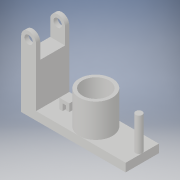
# Autodesk Inventor part: ValveBaseMk2.4
Saved by Autodesk Inventor 2019 (Build 230136000, 136)
## iProperties
Created: 2019-01-19
Part Number: ValveBaseMk2.4
Material: Generic
Document SubType Name: Modeling
Designer: Kepler
Density: 1 g/cm^3
Appearance: Default
Author: Kepler
Autodesk Inventor part; units mm, degrees
ref_plane "YZ Plane" through (0, 0, 0) normal (1, 0, 0) x (0, 1, 0)
ref_plane "XZ Plane" through (0, 0, 0) normal (0, 1, 0) x (-1, 0, 0)
ref_plane "XY Plane" through (0, 0, 0) normal (0, 0, 1) x (1, 0, 0)
sketch "Sketch1" plane through (0, 0, 0) normal (0, 0, 1) x (1, 0, 0)
  line L0 (0, 0) -> (0, 40)
  line L1 (0, 0) -> (63, 0)
  line L2 (63, 0) -> (63, 5)
  line L3 (63, 5) -> (9, 5)
  arc A0 (9, 40) -> (0, 40) centre (4.5, 40) ccw
  line L4 (9, 40) -> (9, 5)
  circle A1 centre (4.5, 40) radius 2.5
  dimension "d0" = 40
  dimension "d2" = 5
  dimension "d6" = 4.5
  dimension "d7" = 5
  dimension "d8" = 9
  dimension "d9" = 54
  dimension "d47" = 32.5
  constraints: 10 end point, 3 perpendicular, 2 centre point, 2 point on circle, 2 tangent, 1 coincident, 1 horizontal, 1 vertical
  measures "d0" distance of L0.start L0.end
  measures "d2" distance of L1.end L2.end
  measures "d6" radius of A0
  measures "d7" diameter of A1
  measures "d8" distance between parallel lines of L4 L0
  measures "d9" distance of L2.end L3.end
  measures "d47" distance edge to line of A1 L3
extrude "Extrusion1" add sketch "Sketch1" along normal blind 20
sketch "Sketch2" plane through (9, 5, 0) normal (0, 1, 0) x (1, 0, 0)
  line L0 (0, 0) -> (0, -20) projected
  circle A0 centre (26, -10) radius 10
  line L1 (0, 0) -> (54, 0) projected
  circle A1 centre (52, -10) radius 2
  line L2 (54, 0) -> (54, -20) projected
  point P0 (-9, 0)
  dimension "d14" = 20
  dimension "d16" = 26
  dimension "d20" = 4
  dimension "d21" = 10
  dimension "d22" = 14
  constraints: 2 centre point, 2 tangent
  measures "d14" diameter of A0
  measures "d16" distance from line of A0.centre L0
  measures "d20" diameter of A1
  measures "d21" distance from line of L1 A1.centre
sketch "Sketch7" plane through (9, 5, 0) normal (1, 0, 0) x (0, 0, -1)
  line L0 (-10, 41.0364) -> (-10, 39.6436)
  line L1 (0, 39.5) -> (-20, 39.5) projected
  line L2 (-2.5, 39.5) -> (-2.5, 25.5)
  line L3 (-17.5, 39.5) -> (-17.5, 25.5)
  line L4 (-17.5, 39.5) -> (-2.5, 39.5)
  line L5 (0, 32.5) -> (-20, 32.5) projected
  line L6 (-17.5, 25.5) -> (-2.5, 25.5)
  point P0 (0, -5)
  dimension "d40" = 14
  dimension "d41" = 14
  dimension "d42" = 15
  constraints: 10 end point, 2 point on line, 2 vertical, 1 collinear, 1 perpendicular, 1 other
  measures "d40" distance of L2.start L2.end
  measures "d41" distance of L3.start L3.end
  measures "d42" distance between parallel lines of L3 L2
extrude "Extrusion5" cut sketch "Sketch7" against normal blind 14
extrude "Extrusion6" add sketch "Sketch2" along normal blind 20
sketch "Sketch9" plane through (35, 25, 10) normal (0, 1, 0) x (1, 0, 0)
  circle A0 centre (0, 0) radius 8
  point P0 (-35, 10)
  dimension "d50" = 16
  constraints: 1 centre point
  measures "d50" diameter of A0
extrude "Extrusion7" cut sketch "Sketch9" against normal blind 25
sketch "Sketch10" plane through (9, 5, 20) normal (0, 1, 0) x (1, 0, 0)
  line L0 (6, 8) -> (12, 8)
  line L1 (12, 8) -> (12, 12)
  line L2 (12, 12) -> (6, 12)
  line L3 (6, 12) -> (6, 8)
  line L4 (26, 0) -> (0, 0) projected
  line L5 (0, 2.5) -> (0, 17.5) projected
  point P0 (-9, 20)
  dimension "d53" = 6
  dimension "d54" = 4
  dimension "d55" = 8
  dimension "d56" = 6
  constraints: 8 end point, 3 perpendicular, 1 horizontal
  measures "d53" distance of L0.start L0.end
  measures "d54" distance of L0.end L1.end
  measures "d55" distance between parallel lines of L4 L0
  measures "d56" distance between parallel lines of L5 L3
extrude "Extrusion8" add sketch "Sketch10" along normal blind 6
sketch "Sketch11" plane through (21, 5, 8) normal (0, 0, -1) x (-1, 0, 0)
  line L0 (2, 4) -> (4, 4)
  line L1 (6, 0) -> (6, 6) projected
  line L2 (12, 0) -> (-14, 0) projected
  line L3 (0, 0) -> (6, 0)
  line L4 (0, 1.5) -> (0, 0)
  line L5 (6, 0) -> (0, 0)
  line L6 (0, 0) -> (3, 0)
  line L7 (0, 1.5) -> (2, 1.5)
  line L8 (2, 1.5) -> (2, 4)
  line L9 (3, 0) -> (0, 0)
  line L10 (4, 4) -> (4, 0)
  line L11 (0, 0) -> (6, 0) projected
  line L12 (0, 0) -> (4, 0)
  point P0 (21, -5)
  dimension "d59" = 2
  dimension "d60" = 2
  dimension "d61" = 4
  dimension "d62" = 1.5
  constraints: 20 end point, 3 perpendicular, 2 horizontal, 1 point on line, 1 vertical
  measures "d59" distance from line of L1 L0.end
  measures "d60" distance of L0.start L0.end
  measures "d61" distance between parallel lines of L2 L0
  measures "d62" distance of L4.start L3.start
extrude "Extrusion9" cut sketch "Sketch11" against normal blind 4
equation "\"d21\" = d19"
equation "\"d40\" = d41"
equation "\"d19\" = 0.5 * d14"
body "Solid1"
